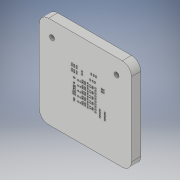
# Autodesk Inventor part: stencil-plate
Saved by Autodesk Inventor 2019.3 (Build 233278000, 278)
## iProperties
Created: 2019-02-09
Part Number: stencil-plate
Material: Generic
Document SubType Name: Modeling
Designer: mark
Density: 1 g/cm^3
Appearance: Default
Author: mark
Autodesk Inventor part; units mm, degrees
ref_plane "YZ Plane" through (0, 0, 0) normal (1, 0, 0) x (0, 1, 0)
ref_plane "XZ Plane" through (0, 0, 0) normal (0, 1, 0) x (-1, 0, 0)
ref_plane "XY Plane" through (0, 0, 0) normal (0, 0, 1) x (1, 0, 0)
sketch "Sketch1" plane through (0, 0, 0) normal (0, 0, 1) x (1, 0, 0)
  line L0 (91.0856, -138.6977) -> (191.0856, -138.6977)
  line L1 (191.0856, -138.6977) -> (191.0856, -38.6977)
  line L2 (191.0856, -38.6977) -> (91.0856, -38.6977)
  line L3 (91.0856, -38.6977) -> (91.0856, -138.6977)
  circle A0 centre (105.0001, -55.0001) radius 2.62
  circle A1 centre (175.0003, -55.0001) radius 2.6201
  line L4 (157.55, -104.61) -> (156.05, -104.61)
  line L5 (156.05, -104.61) -> (156.05, -104.01)
  line L6 (156.05, -104.01) -> (157.55, -104.01)
  line L7 (157.55, -104.01) -> (157.55, -104.61)
  line L8 (162.95, -104.61) -> (161.45, -104.61)
  line L9 (161.45, -104.61) -> (161.45, -104.01)
  line L10 (161.45, -104.01) -> (162.95, -104.01)
  line L11 (162.95, -104.01) -> (162.95, -104.61)
  line L12 (157.55, -103.34) -> (156.05, -103.34)
  line L13 (156.05, -103.34) -> (156.05, -102.74)
  line L14 (156.05, -102.74) -> (157.55, -102.74)
  line L15 (157.55, -102.74) -> (157.55, -103.34)
  line L16 (162.95, -103.34) -> (161.45, -103.34)
  line L17 (161.45, -103.34) -> (161.45, -102.74)
  line L18 (161.45, -102.74) -> (162.95, -102.74)
  line L19 (162.95, -102.74) -> (162.95, -103.34)
  line L20 (129.8, -102.505) -> (128.2, -102.505)
  line L21 (128.2, -102.505) -> (128.2, -101.255)
  line L22 (128.2, -101.255) -> (129.8, -101.255)
  line L23 (129.8, -101.255) -> (129.8, -102.505)
  line L24 (152.625, -102.5) -> (151.375, -102.5)
  line L25 (151.375, -102.5) -> (151.375, -101)
  line L26 (151.375, -101) -> (152.625, -101)
  line L27 (152.625, -101) -> (152.625, -102.5)
  line L28 (144.15, -102.1) -> (142.85, -102.1)
  line L29 (142.85, -102.1) -> (142.85, -100.6)
  line L30 (142.85, -100.6) -> (144.15, -100.6)
  line L31 (144.15, -100.6) -> (144.15, -102.1)
  line L32 (162.95, -102.07) -> (161.45, -102.07)
  line L33 (161.45, -102.07) -> (161.45, -101.47)
  line L34 (161.45, -101.47) -> (162.95, -101.47)
  line L35 (162.95, -101.47) -> (162.95, -102.07)
  line L36 (157.55, -102.07) -> (156.05, -102.07)
  line L37 (156.05, -102.07) -> (156.05, -101.47)
  line L38 (156.05, -101.47) -> (157.55, -101.47)
  line L39 (157.55, -101.47) -> (157.55, -102.07)
  line L40 (136.6, -101.65) -> (135.1, -101.65)
  line L41 (135.1, -101.65) -> (135.1, -100.35)
  line L42 (135.1, -100.35) -> (136.6, -100.35)
  line L43 (136.6, -100.35) -> (136.6, -101.65)
  line L44 (133.9, -101.65) -> (132.4, -101.65)
  line L45 (132.4, -101.65) -> (132.4, -100.35)
  line L46 (132.4, -100.35) -> (133.9, -100.35)
  line L47 (133.9, -100.35) -> (133.9, -101.65)
  line L48 (141.5, -101.625) -> (140, -101.625)
  line L49 (140, -101.625) -> (140, -100.375)
  line L50 (140, -100.375) -> (141.5, -100.375)
  line L51 (141.5, -100.375) -> (141.5, -101.625)
  line L52 (139, -101.625) -> (137.5, -101.625)
  line L53 (137.5, -101.625) -> (137.5, -100.375)
  line L54 (137.5, -100.375) -> (139, -100.375)
  line L55 (139, -100.375) -> (139, -101.625)
  line L56 (146.93, -101.275) -> (145.37, -101.275)
  line L57 (145.37, -101.275) -> (145.37, -100.625)
  line L58 (145.37, -100.625) -> (146.93, -100.625)
  line L59 (146.93, -100.625) -> (146.93, -101.275)
  line L60 (149.63, -101.275) -> (148.07, -101.275)
  line L61 (148.07, -101.275) -> (148.07, -100.625)
  line L62 (148.07, -100.625) -> (149.63, -100.625)
  line L63 (149.63, -100.625) -> (149.63, -101.275)
  line L64 (162.95, -100.8) -> (161.45, -100.8)
  line L65 (161.45, -100.8) -> (161.45, -100.2)
  line L66 (161.45, -100.2) -> (162.95, -100.2)
  line L67 (162.95, -100.2) -> (162.95, -100.8)
  line L68 (157.55, -100.8) -> (156.05, -100.8)
  line L69 (156.05, -100.8) -> (156.05, -100.2)
  line L70 (156.05, -100.2) -> (157.55, -100.2)
  line L71 (157.55, -100.2) -> (157.55, -100.8)
  line L72 (129.8, -100.745) -> (128.2, -100.745)
  line L73 (128.2, -100.745) -> (128.2, -99.495)
  line L74 (128.2, -99.495) -> (129.8, -99.495)
  line L75 (129.8, -99.495) -> (129.8, -100.745)
  line L76 (149.63, -100.325) -> (148.07, -100.325)
  line L77 (148.07, -100.325) -> (148.07, -99.675)
  line L78 (148.07, -99.675) -> (149.63, -99.675)
  line L79 (149.63, -99.675) -> (149.63, -100.325)
  line L80 (152.625, -100) -> (151.375, -100)
  line L81 (151.375, -100) -> (151.375, -98.5)
  line L82 (151.375, -98.5) -> (152.625, -98.5)
  line L83 (152.625, -98.5) -> (152.625, -100)
  line L84 (141.6, -99.65) -> (140.1, -99.65)
  line L85 (140.1, -99.65) -> (140.1, -98.35)
  line L86 (140.1, -98.35) -> (141.6, -98.35)
  line L87 (141.6, -98.35) -> (141.6, -99.65)
  line L88 (138.9, -99.65) -> (137.4, -99.65)
  line L89 (137.4, -99.65) -> (137.4, -98.35)
  line L90 (137.4, -98.35) -> (138.9, -98.35)
  line L91 (138.9, -98.35) -> (138.9, -99.65)
  line L92 (162.95, -99.53) -> (161.45, -99.53)
  line L93 (161.45, -99.53) -> (161.45, -98.93)
  line L94 (161.45, -98.93) -> (162.95, -98.93)
  line L95 (162.95, -98.93) -> (162.95, -99.53)
  line L96 (157.55, -99.53) -> (156.05, -99.53)
  line L97 (156.05, -99.53) -> (156.05, -98.93)
  line L98 (156.05, -98.93) -> (157.55, -98.93)
  line L99 (157.55, -98.93) -> (157.55, -99.53)
  line L100 (144.15, -99.4) -> (142.85, -99.4)
  line L101 (142.85, -99.4) -> (142.85, -97.9)
  line L102 (142.85, -97.9) -> (144.15, -97.9)
  line L103 (144.15, -97.9) -> (144.15, -99.4)
  line L104 (146.93, -99.375) -> (145.37, -99.375)
  line L105 (145.37, -99.375) -> (145.37, -98.725)
  line L106 (145.37, -98.725) -> (146.93, -98.725)
  line L107 (146.93, -98.725) -> (146.93, -99.375)
  line L108 (149.63, -99.375) -> (148.07, -99.375)
  line L109 (148.07, -99.375) -> (148.07, -98.725)
  line L110 (148.07, -98.725) -> (149.63, -98.725)
  line L111 (149.63, -98.725) -> (149.63, -99.375)
  line L112 (157.55, -98.26) -> (156.05, -98.26)
  line L113 (156.05, -98.26) -> (156.05, -97.66)
  line L114 (156.05, -97.66) -> (157.55, -97.66)
  line L115 (157.55, -97.66) -> (157.55, -98.26)
  line L116 (162.95, -98.26) -> (161.45, -98.26)
  line L117 (161.45, -98.26) -> (161.45, -97.66)
  line L118 (161.45, -97.66) -> (162.95, -97.66)
  line L119 (162.95, -97.66) -> (162.95, -98.26)
  line L120 (152.625, -97.5) -> (151.375, -97.5)
  line L121 (151.375, -97.5) -> (151.375, -96)
  line L122 (151.375, -96) -> (152.625, -96)
  line L123 (152.625, -96) -> (152.625, -97.5)
  line L124 (144.15, -97.1) -> (142.85, -97.1)
  line L125 (142.85, -97.1) -> (142.85, -95.6)
  line L126 (142.85, -95.6) -> (144.15, -95.6)
  line L127 (144.15, -95.6) -> (144.15, -97.1)
  line L128 (157.55, -96.99) -> (156.05, -96.99)
  line L129 (156.05, -96.99) -> (156.05, -96.39)
  line L130 (156.05, -96.39) -> (157.55, -96.39)
  line L131 (157.55, -96.39) -> (157.55, -96.99)
  line L132 (162.95, -96.99) -> (161.45, -96.99)
  line L133 (161.45, -96.99) -> (161.45, -96.39)
  line L134 (161.45, -96.39) -> (162.95, -96.39)
  line L135 (162.95, -96.39) -> (162.95, -96.99)
  line L136 (130.65, -96.7) -> (127.35, -96.7)
  line L137 (127.35, -96.7) -> (127.35, -96.2)
  line L138 (127.35, -96.2) -> (130.65, -96.2)
  line L139 (130.65, -96.2) -> (130.65, -96.7)
  line L140 (133.9, -96.65) -> (132.4, -96.65)
  line L141 (132.4, -96.65) -> (132.4, -95.35)
  line L142 (132.4, -95.35) -> (133.9, -95.35)
  line L143 (133.9, -95.35) -> (133.9, -96.65)
  line L144 (136.6, -96.65) -> (135.1, -96.65)
  line L145 (135.1, -96.65) -> (135.1, -95.35)
  line L146 (135.1, -95.35) -> (136.6, -95.35)
  line L147 (136.6, -95.35) -> (136.6, -96.65)
  line L148 (139, -96.625) -> (137.5, -96.625)
  line L149 (137.5, -96.625) -> (137.5, -95.375)
  line L150 (137.5, -95.375) -> (139, -95.375)
  line L151 (139, -95.375) -> (139, -96.625)
  line L152 (141.5, -96.625) -> (140, -96.625)
  line L153 (140, -96.625) -> (140, -95.375)
  line L154 (140, -95.375) -> (141.5, -95.375)
  line L155 (141.5, -95.375) -> (141.5, -96.625)
  line L156 (146.93, -96.275) -> (145.37, -96.275)
  line L157 (145.37, -96.275) -> (145.37, -95.625)
  line L158 (145.37, -95.625) -> (146.93, -95.625)
  line L159 (146.93, -95.625) -> (146.93, -96.275)
  line L160 (149.63, -96.275) -> (148.07, -96.275)
  line L161 (148.07, -96.275) -> (148.07, -95.625)
  line L162 (148.07, -95.625) -> (149.63, -95.625)
  line L163 (149.63, -95.625) -> (149.63, -96.275)
  line L164 (130.65, -95.65) -> (127.35, -95.65)
  line L165 (127.35, -95.65) -> (127.35, -94.35)
  line L166 (127.35, -94.35) -> (130.65, -94.35)
  line L167 (130.65, -94.35) -> (130.65, -95.65)
  line L168 (149.63, -95.325) -> (148.07, -95.325)
  line L169 (148.07, -95.325) -> (148.07, -94.675)
  line L170 (148.07, -94.675) -> (149.63, -94.675)
  line L171 (149.63, -94.675) -> (149.63, -95.325)
  line L172 (152.625, -95) -> (151.375, -95)
  line L173 (151.375, -95) -> (151.375, -93.5)
  line L174 (151.375, -93.5) -> (152.625, -93.5)
  line L175 (152.625, -93.5) -> (152.625, -95)
  line L176 (138.9, -94.65) -> (137.4, -94.65)
  line L177 (137.4, -94.65) -> (137.4, -93.35)
  line L178 (137.4, -93.35) -> (138.9, -93.35)
  line L179 (138.9, -93.35) -> (138.9, -94.65)
  line L180 (141.6, -94.65) -> (140.1, -94.65)
  line L181 (140.1, -94.65) -> (140.1, -93.35)
  line L182 (140.1, -93.35) -> (141.6, -93.35)
  line L183 (141.6, -93.35) -> (141.6, -94.65)
  line L184 (144.15, -94.4) -> (142.85, -94.4)
  line L185 (142.85, -94.4) -> (142.85, -92.9)
  line L186 (142.85, -92.9) -> (144.15, -92.9)
  line L187 (144.15, -92.9) -> (144.15, -94.4)
  line L188 (146.93, -94.375) -> (145.37, -94.375)
  line L189 (145.37, -94.375) -> (145.37, -93.725)
  line L190 (145.37, -93.725) -> (146.93, -93.725)
  line L191 (146.93, -93.725) -> (146.93, -94.375)
  line L192 (149.63, -94.375) -> (148.07, -94.375)
  line L193 (148.07, -94.375) -> (148.07, -93.725)
  line L194 (148.07, -93.725) -> (149.63, -93.725)
  line L195 (149.63, -93.725) -> (149.63, -94.375)
  line L196 (130.65, -93.8) -> (127.35, -93.8)
  line L197 (127.35, -93.8) -> (127.35, -93.3)
  line L198 (127.35, -93.3) -> (130.65, -93.3)
  line L199 (130.65, -93.3) -> (130.65, -93.8)
  line L200 (152.625, -92.5) -> (151.375, -92.5)
  line L201 (151.375, -92.5) -> (151.375, -91)
  line L202 (151.375, -91) -> (152.625, -91)
  line L203 (152.625, -91) -> (152.625, -92.5)
  line L204 (130.35, -92.3) -> (127.65, -92.3)
  line L205 (127.65, -92.3) -> (127.65, -90.9)
  line L206 (127.65, -90.9) -> (130.35, -90.9)
  line L207 (130.35, -90.9) -> (130.35, -92.3)
  line L208 (144.15, -92.1) -> (142.85, -92.1)
  line L209 (142.85, -92.1) -> (142.85, -90.6)
  line L210 (142.85, -90.6) -> (144.15, -90.6)
  line L211 (144.15, -90.6) -> (144.15, -92.1)
  line L212 (133.9, -91.65) -> (132.4, -91.65)
  line L213 (132.4, -91.65) -> (132.4, -90.35)
  line L214 (132.4, -90.35) -> (133.9, -90.35)
  line L215 (133.9, -90.35) -> (133.9, -91.65)
  line L216 (136.6, -91.65) -> (135.1, -91.65)
  line L217 (135.1, -91.65) -> (135.1, -90.35)
  line L218 (135.1, -90.35) -> (136.6, -90.35)
  line L219 (136.6, -90.35) -> (136.6, -91.65)
  line L220 (141.5, -91.625) -> (140, -91.625)
  line L221 (140, -91.625) -> (140, -90.375)
  line L222 (140, -90.375) -> (141.5, -90.375)
  line L223 (141.5, -90.375) -> (141.5, -91.625)
  line L224 (139, -91.625) -> (137.5, -91.625)
  line L225 (137.5, -91.625) -> (137.5, -90.375)
  line L226 (137.5, -90.375) -> (139, -90.375)
  line L227 (139, -90.375) -> (139, -91.625)
  line L228 (149.63, -91.275) -> (148.07, -91.275)
  line L229 (148.07, -91.275) -> (148.07, -90.625)
  line L230 (148.07, -90.625) -> (149.63, -90.625)
  line L231 (149.63, -90.625) -> (149.63, -91.275)
  line L232 (146.93, -91.275) -> (145.37, -91.275)
  line L233 (145.37, -91.275) -> (145.37, -90.625)
  line L234 (145.37, -90.625) -> (146.93, -90.625)
  line L235 (146.93, -90.625) -> (146.93, -91.275)
  line L236 (149.63, -90.325) -> (148.07, -90.325)
  line L237 (148.07, -90.325) -> (148.07, -89.675)
  line L238 (148.07, -89.675) -> (149.63, -89.675)
  line L239 (149.63, -89.675) -> (149.63, -90.325)
  line L240 (130.35, -90.15) -> (127.65, -90.15)
  line L241 (127.65, -90.15) -> (127.65, -87.65)
  line L242 (127.65, -87.65) -> (130.35, -87.65)
  line L243 (130.35, -87.65) -> (130.35, -90.15)
  line L244 (152.625, -90) -> (151.375, -90)
  line L245 (151.375, -90) -> (151.375, -88.5)
  line L246 (151.375, -88.5) -> (152.625, -88.5)
  line L247 (152.625, -88.5) -> (152.625, -90)
  line L248 (138.9, -89.65) -> (137.4, -89.65)
  line L249 (137.4, -89.65) -> (137.4, -88.35)
  line L250 (137.4, -88.35) -> (138.9, -88.35)
  line L251 (138.9, -88.35) -> (138.9, -89.65)
  line L252 (141.6, -89.65) -> (140.1, -89.65)
  line L253 (140.1, -89.65) -> (140.1, -88.35)
  line L254 (140.1, -88.35) -> (141.6, -88.35)
  line L255 (141.6, -88.35) -> (141.6, -89.65)
  line L256 (144.15, -89.4) -> (142.85, -89.4)
  line L257 (142.85, -89.4) -> (142.85, -87.9)
  line L258 (142.85, -87.9) -> (144.15, -87.9)
  line L259 (144.15, -87.9) -> (144.15, -89.4)
  line L260 (146.93, -89.375) -> (145.37, -89.375)
  line L261 (145.37, -89.375) -> (145.37, -88.725)
  line L262 (145.37, -88.725) -> (146.93, -88.725)
  line L263 (146.93, -88.725) -> (146.93, -89.375)
  line L264 (149.63, -89.375) -> (148.07, -89.375)
  line L265 (148.07, -89.375) -> (148.07, -88.725)
  line L266 (148.07, -88.725) -> (149.63, -88.725)
  line L267 (149.63, -88.725) -> (149.63, -89.375)
  line L268 (152.625, -87.5) -> (151.375, -87.5)
  line L269 (151.375, -87.5) -> (151.375, -86)
  line L270 (151.375, -86) -> (152.625, -86)
  line L271 (152.625, -86) -> (152.625, -87.5)
  line L272 (144.15, -87.1) -> (142.85, -87.1)
  line L273 (142.85, -87.1) -> (142.85, -85.6)
  line L274 (142.85, -85.6) -> (144.15, -85.6)
  line L275 (144.15, -85.6) -> (144.15, -87.1)
  line L276 (133.9, -86.65) -> (132.4, -86.65)
  line L277 (132.4, -86.65) -> (132.4, -85.35)
  line L278 (132.4, -85.35) -> (133.9, -85.35)
  line L279 (133.9, -85.35) -> (133.9, -86.65)
  line L280 (136.6, -86.65) -> (135.1, -86.65)
  line L281 (135.1, -86.65) -> (135.1, -85.35)
  line L282 (135.1, -85.35) -> (136.6, -85.35)
  line L283 (136.6, -85.35) -> (136.6, -86.65)
  line L284 (141.5, -86.625) -> (140, -86.625)
  line L285 (140, -86.625) -> (140, -85.375)
  line L286 (140, -85.375) -> (141.5, -85.375)
  line L287 (141.5, -85.375) -> (141.5, -86.625)
  line L288 (139, -86.625) -> (137.5, -86.625)
  line L289 (137.5, -86.625) -> (137.5, -85.375)
  line L290 (137.5, -85.375) -> (139, -85.375)
  line L291 (139, -85.375) -> (139, -86.625)
  line L292 (146.93, -86.275) -> (145.37, -86.275)
  line L293 (145.37, -86.275) -> (145.37, -85.625)
  line L294 (145.37, -85.625) -> (146.93, -85.625)
  line L295 (146.93, -85.625) -> (146.93, -86.275)
  line L296 (149.63, -86.275) -> (148.07, -86.275)
  line L297 (148.07, -86.275) -> (148.07, -85.625)
  line L298 (148.07, -85.625) -> (149.63, -85.625)
  line L299 (149.63, -85.625) -> (149.63, -86.275)
  line L300 (129.8, -86.265) -> (128.2, -86.265)
  line L301 (128.2, -86.265) -> (128.2, -85.615)
  line L302 (128.2, -85.615) -> (129.8, -85.615)
  line L303 (129.8, -85.615) -> (129.8, -86.265)
  line L304 (129.8, -85.325) -> (128.2, -85.325)
  line L305 (128.2, -85.325) -> (128.2, -84.675)
  line L306 (128.2, -84.675) -> (129.8, -84.675)
  line L307 (129.8, -84.675) -> (129.8, -85.325)
  line L308 (149.63, -85.325) -> (148.07, -85.325)
  line L309 (148.07, -85.325) -> (148.07, -84.675)
  line L310 (148.07, -84.675) -> (149.63, -84.675)
  line L311 (149.63, -84.675) -> (149.63, -85.325)
  line L312 (152.625, -85) -> (151.375, -85)
  line L313 (151.375, -85) -> (151.375, -83.5)
  line L314 (151.375, -83.5) -> (152.625, -83.5)
  line L315 (152.625, -83.5) -> (152.625, -85)
  line L316 (141.6, -84.65) -> (140.1, -84.65)
  line L317 (140.1, -84.65) -> (140.1, -83.35)
  line L318 (140.1, -83.35) -> (141.6, -83.35)
  line L319 (141.6, -83.35) -> (141.6, -84.65)
  line L320 (138.9, -84.65) -> (137.4, -84.65)
  line L321 (137.4, -84.65) -> (137.4, -83.35)
  line L322 (137.4, -83.35) -> (138.9, -83.35)
  line L323 (138.9, -83.35) -> (138.9, -84.65)
  line L324 (144.15, -84.4) -> (142.85, -84.4)
  line L325 (142.85, -84.4) -> (142.85, -82.9)
  line L326 (142.85, -82.9) -> (144.15, -82.9)
  line L327 (144.15, -82.9) -> (144.15, -84.4)
  line L328 (149.63, -84.375) -> (148.07, -84.375)
  line L329 (148.07, -84.375) -> (148.07, -83.725)
  line L330 (148.07, -83.725) -> (149.63, -83.725)
  line L331 (149.63, -83.725) -> (149.63, -84.375)
  line L332 (146.93, -84.375) -> (145.37, -84.375)
  line L333 (145.37, -84.375) -> (145.37, -83.725)
  line L334 (145.37, -83.725) -> (146.93, -83.725)
  line L335 (146.93, -83.725) -> (146.93, -84.375)
  line L336 (152.625, -82.5) -> (151.375, -82.5)
  line L337 (151.375, -82.5) -> (151.375, -81)
  line L338 (151.375, -81) -> (152.625, -81)
  line L339 (152.625, -81) -> (152.625, -82.5)
  line L340 (144.15, -82.1) -> (142.85, -82.1)
  line L341 (142.85, -82.1) -> (142.85, -80.6)
  line L342 (142.85, -80.6) -> (144.15, -80.6)
  line L343 (144.15, -80.6) -> (144.15, -82.1)
  line L344 (133.9, -81.65) -> (132.4, -81.65)
  line L345 (132.4, -81.65) -> (132.4, -80.35)
  line L346 (132.4, -80.35) -> (133.9, -80.35)
  line L347 (133.9, -80.35) -> (133.9, -81.65)
  line L348 (136.6, -81.65) -> (135.1, -81.65)
  line L349 (135.1, -81.65) -> (135.1, -80.35)
  line L350 (135.1, -80.35) -> (136.6, -80.35)
  line L351 (136.6, -80.35) -> (136.6, -81.65)
  line L352 (139, -81.625) -> (137.5, -81.625)
  line L353 (137.5, -81.625) -> (137.5, -80.375)
  line L354 (137.5, -80.375) -> (139, -80.375)
  line L355 (139, -80.375) -> (139, -81.625)
  line L356 (141.5, -81.625) -> (140, -81.625)
  line L357 (140, -81.625) -> (140, -80.375)
  line L358 (140, -80.375) -> (141.5, -80.375)
  line L359 (141.5, -80.375) -> (141.5, -81.625)
  line L360 (129.8, -81.325) -> (128.2, -81.325)
  line L361 (128.2, -81.325) -> (128.2, -80.675)
  line L362 (128.2, -80.675) -> (129.8, -80.675)
  line L363 (129.8, -80.675) -> (129.8, -81.325)
  line L364 (146.93, -81.275) -> (145.37, -81.275)
  line L365 (145.37, -81.275) -> (145.37, -80.625)
  line L366 (145.37, -80.625) -> (146.93, -80.625)
  line L367 (146.93, -80.625) -> (146.93, -81.275)
  line L368 (149.63, -81.275) -> (148.07, -81.275)
  line L369 (148.07, -81.275) -> (148.07, -80.625)
  line L370 (148.07, -80.625) -> (149.63, -80.625)
  line L371 (149.63, -80.625) -> (149.63, -81.275)
  line L372 (129.8, -80.385) -> (128.2, -80.385)
  line L373 (128.2, -80.385) -> (128.2, -79.735)
  line L374 (128.2, -79.735) -> (129.8, -79.735)
  line L375 (129.8, -79.735) -> (129.8, -80.385)
  line L376 (149.63, -80.325) -> (148.07, -80.325)
  line L377 (148.07, -80.325) -> (148.07, -79.675)
  line L378 (148.07, -79.675) -> (149.63, -79.675)
  line L379 (149.63, -79.675) -> (149.63, -80.325)
  line L380 (152.625, -80) -> (151.375, -80)
  line L381 (151.375, -80) -> (151.375, -78.5)
  line L382 (151.375, -78.5) -> (152.625, -78.5)
  line L383 (152.625, -78.5) -> (152.625, -80)
  line L384 (161.375, -79.75) -> (160.125, -79.75)
  line L385 (160.125, -79.75) -> (160.125, -78.25)
  line L386 (160.125, -78.25) -> (161.375, -78.25)
  line L387 (161.375, -78.25) -> (161.375, -79.75)
  line L388 (159.375, -79.75) -> (158.125, -79.75)
  line L389 (158.125, -79.75) -> (158.125, -78.25)
  line L390 (158.125, -78.25) -> (159.375, -78.25)
  line L391 (159.375, -78.25) -> (159.375, -79.75)
  line L392 (141.6, -79.65) -> (140.1, -79.65)
  line L393 (140.1, -79.65) -> (140.1, -78.35)
  line L394 (140.1, -78.35) -> (141.6, -78.35)
  line L395 (141.6, -78.35) -> (141.6, -79.65)
  line L396 (138.9, -79.65) -> (137.4, -79.65)
  line L397 (137.4, -79.65) -> (137.4, -78.35)
  line L398 (137.4, -78.35) -> (138.9, -78.35)
  line L399 (138.9, -78.35) -> (138.9, -79.65)
  line L400 (144.15, -79.4) -> (142.85, -79.4)
  line L401 (142.85, -79.4) -> (142.85, -77.9)
  line L402 (142.85, -77.9) -> (144.15, -77.9)
  line L403 (144.15, -77.9) -> (144.15, -79.4)
  line L404 (146.93, -79.375) -> (145.37, -79.375)
  line L405 (145.37, -79.375) -> (145.37, -78.725)
  line L406 (145.37, -78.725) -> (146.93, -78.725)
  line L407 (146.93, -78.725) -> (146.93, -79.375)
  line L408 (149.63, -79.375) -> (148.07, -79.375)
  line L409 (148.07, -79.375) -> (148.07, -78.725)
  line L410 (148.07, -78.725) -> (149.63, -78.725)
  line L411 (149.63, -78.725) -> (149.63, -79.375)
  line L412 (159.375, -77.25) -> (158.125, -77.25)
  line L413 (158.125, -77.25) -> (158.125, -75.75)
  line L414 (158.125, -75.75) -> (159.375, -75.75)
  line L415 (159.375, -75.75) -> (159.375, -77.25)
  line L416 (161.375, -77.25) -> (160.125, -77.25)
  line L417 (160.125, -77.25) -> (160.125, -75.75)
  line L418 (160.125, -75.75) -> (161.375, -75.75)
  line L419 (161.375, -75.75) -> (161.375, -77.25)
  line L420 (132.04, -76.1) -> (131.04, -76.1)
  line L421 (131.04, -76.1) -> (131.04, -72.95)
  line L422 (131.04, -72.95) -> (132.04, -72.95)
  line L423 (132.04, -72.95) -> (132.04, -76.1)
  line L424 (129.5, -76.1) -> (128.5, -76.1)
  line L425 (128.5, -76.1) -> (128.5, -72.95)
  line L426 (128.5, -72.95) -> (129.5, -72.95)
  line L427 (129.5, -72.95) -> (129.5, -76.1)
  line L428 (126.96, -76.1) -> (125.96, -76.1)
  line L429 (125.96, -76.1) -> (125.96, -72.95)
  line L430 (125.96, -72.95) -> (126.96, -72.95)
  line L431 (126.96, -72.95) -> (126.96, -76.1)
  line L432 (152.01, -75) -> (150.81, -75)
  line L433 (150.81, -75) -> (150.81, -73)
  line L434 (150.81, -73) -> (152.01, -73)
  line L435 (152.01, -73) -> (152.01, -75)
  line L436 (149.47, -75) -> (148.27, -75)
  line L437 (148.27, -75) -> (148.27, -73)
  line L438 (148.27, -73) -> (149.47, -73)
  line L439 (149.47, -73) -> (149.47, -75)
  line L440 (146.93, -75) -> (145.73, -75)
  line L441 (145.73, -75) -> (145.73, -73)
  line L442 (145.73, -73) -> (146.93, -73)
  line L443 (146.93, -73) -> (146.93, -75)
  line L444 (138.15, -74.1) -> (136.85, -74.1)
  line L445 (136.85, -74.1) -> (136.85, -72.6)
  line L446 (136.85, -72.6) -> (138.15, -72.6)
  line L447 (138.15, -72.6) -> (138.15, -74.1)
  line L448 (138.15, -71.4) -> (136.85, -71.4)
  line L449 (136.85, -71.4) -> (136.85, -69.9)
  line L450 (136.85, -69.9) -> (138.15, -69.9)
  line L451 (138.15, -69.9) -> (138.15, -71.4)
  line L452 (132.04, -71.05) -> (131.04, -71.05)
  line L453 (131.04, -71.05) -> (131.04, -67.9)
  line L454 (131.04, -67.9) -> (132.04, -67.9)
  line L455 (132.04, -67.9) -> (132.04, -71.05)
  line L456 (129.5, -71.05) -> (128.5, -71.05)
  line L457 (128.5, -71.05) -> (128.5, -67.9)
  line L458 (128.5, -67.9) -> (129.5, -67.9)
  line L459 (129.5, -67.9) -> (129.5, -71.05)
  line L460 (126.96, -71.05) -> (125.96, -71.05)
  line L461 (125.96, -71.05) -> (125.96, -67.9)
  line L462 (125.96, -67.9) -> (126.96, -67.9)
  line L463 (126.96, -67.9) -> (126.96, -71.05)
  line L464 (153.28, -69) -> (152.08, -69)
  line L465 (152.08, -69) -> (152.08, -67)
  line L466 (152.08, -67) -> (153.28, -67)
  line L467 (153.28, -67) -> (153.28, -69)
  line L468 (150.74, -69) -> (149.54, -69)
  line L469 (149.54, -69) -> (149.54, -67)
  line L470 (149.54, -67) -> (150.74, -67)
  line L471 (150.74, -67) -> (150.74, -69)
  line L472 (148.2, -69) -> (147, -69)
  line L473 (147, -69) -> (147, -67)
  line L474 (147, -67) -> (148.2, -67)
  line L475 (148.2, -67) -> (148.2, -69)
  dimension "d0" = 100
  dimension "d1" = 100
  constraints: 952 end point, 2 centre point, 1 perpendicular
  measures "d0" distance between parallel lines of L1 L3
  measures "d1" distance between parallel lines of L0 L2
extrude "Extrusion4" add sketch "Sketch1" along normal blind 10
fillet "Fillet2" radius 10 4 edges at (191.0856, -38.6977, 5) (191.0856, -138.6977, 5) (91.0856, -38.6977, 5) (91.0856, -138.6977, 5)
body "Solid2"
